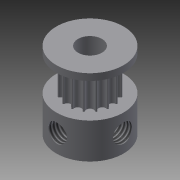
# Autodesk Inventor part: Pulley
Saved by Autodesk Inventor 2015 (Build 190159000, 159)
## iProperties
Created: 2017-01-19
Part Number: Pulley
Material: Generic
Document SubType Name: Modeling
Designer: Ernest
Density: 1 g/cm^3
Appearance: Default
Mass: 1.3342 g
Surface Area: 14.8455 cm^2
Volume: 1.3342 cm^3
Author: Ernest
Autodesk Inventor part; units mm, degrees
ref_plane "YZ Plane" through (0, 0, 0) normal (1, 0, 0) x (0, 1, 0)
ref_plane "XZ Plane" through (0, 0, 0) normal (0, 1, 0) x (-1, 0, 0)
ref_plane "XY Plane" through (0, 0, 0) normal (0, 0, 1) x (1, 0, 0)
sketch "Sketch1" plane through (0, 0, 0) normal (0, 0, 1) x (1, 0, 0)
  arc A0 (-0.7443, 4.7926) -> (-1.1464, 4.7126) centre (0, 0) ccw
  line L0 (0, 0) -> (0, 4.7) construction
  arc A1 (-0.7443, 4.7926) -> (0.7443, 4.7926) centre (0, 4.7) ccw
  arc A2 (-2.5216, 4.1429) -> (-1.1464, 4.7126) centre (-1.7986, 4.3422) ccw
  arc A3 (-3.9151, 2.8626) -> (-2.8626, 3.9151) centre (-3.3234, 3.3234) ccw
  arc A4 (-4.7126, 1.1464) -> (-4.1429, 2.5216) centre (-4.3422, 1.7986) ccw
  arc A5 (-4.7926, -0.7443) -> (-4.7926, 0.7443) centre (-4.7, 0) ccw
  arc A6 (-4.1429, -2.5216) -> (-4.7126, -1.1464) centre (-4.3422, -1.7986) ccw
  arc A7 (-2.8626, -3.9151) -> (-3.9151, -2.8626) centre (-3.3234, -3.3234) ccw
  arc A8 (-1.1464, -4.7126) -> (-2.5216, -4.1429) centre (-1.7986, -4.3422) ccw
  arc A9 (0.7443, -4.7926) -> (-0.7443, -4.7926) centre (0, -4.7) ccw
  arc A10 (2.5216, -4.1429) -> (1.1464, -4.7126) centre (1.7986, -4.3422) ccw
  arc A11 (3.9151, -2.8626) -> (2.8626, -3.9151) centre (3.3234, -3.3234) ccw
  arc A12 (4.7126, -1.1464) -> (4.1429, -2.5216) centre (4.3422, -1.7986) ccw
  arc A13 (4.7926, 0.7443) -> (4.7926, -0.7443) centre (4.7, 0) ccw
  arc A14 (4.1429, 2.5216) -> (4.7126, 1.1464) centre (4.3422, 1.7986) ccw
  arc A15 (2.8626, 3.9151) -> (3.9151, 2.8626) centre (3.3234, 3.3234) ccw
  arc A16 (1.1464, 4.7126) -> (2.5216, 4.1429) centre (1.7986, 4.3422) ccw
  arc A17 (1.1464, 4.7126) -> (0.7443, 4.7926) centre (0, 0) ccw
  arc A18 (2.8626, 3.9151) -> (2.5216, 4.1429) centre (0, 0) ccw
  arc A19 (4.1429, 2.5216) -> (3.9151, 2.8626) centre (0, 0) ccw
  arc A20 (4.7926, 0.7443) -> (4.7126, 1.1464) centre (0, 0) ccw
  arc A21 (4.7126, -1.1464) -> (4.7926, -0.7443) centre (0, 0) ccw
  arc A22 (3.9151, -2.8626) -> (4.1429, -2.5216) centre (0, 0) ccw
  arc A23 (2.5216, -4.1429) -> (2.8626, -3.9151) centre (0, 0) ccw
  arc A24 (0.7443, -4.7926) -> (1.1464, -4.7126) centre (0, 0) ccw
  arc A25 (0, -4.85) -> (0.7443, -4.7926) centre (0, 0) ccw
  arc A26 (-1.1464, -4.7126) -> (-0.7443, -4.7926) centre (0, 0) ccw
  arc A27 (-2.8626, -3.9151) -> (-2.5216, -4.1429) centre (0, 0) ccw
  arc A28 (-4.1429, -2.5216) -> (-3.9151, -2.8626) centre (0, 0) ccw
  arc A29 (-4.7926, -0.7443) -> (-4.7126, -1.1464) centre (0, 0) ccw
  arc A30 (-4.7126, 1.1464) -> (-4.7926, 0.7443) centre (0, 0) ccw
  arc A31 (-3.9151, 2.8626) -> (-4.1429, 2.5216) centre (0, 0) ccw
  arc A32 (-2.5216, 4.1429) -> (-2.8626, 3.9151) centre (0, 0) ccw
  dimension "d0" = 9.7
  dimension "d1" = 4.7
  dimension "d2" = 1.5
  dimension "d5" = 360
  constraints: 66 point on circle, 33 centre point, 2 coincident, 2 end point, 1 point on line, 1 vertical, 65 other
  measures "d0" diameter of A0
  measures "d1" distance of L0.start L0.end
  measures "d2" diameter of A1
extrude "Extrusion1" add sketch "Sketch1" along normal blind 7.15
fillet "Fillet1" radius 0.14 32 edges at (-0.7443, 4.7926, 3.575) (-1.1464, 4.7126, 3.575) (0.7443, 4.7926, 3.575) (1.1464, 4.7126, 3.575) (2.5216, 4.1429, 3.575) (2.8626, 3.9151, 3.575) (-2.5216, 4.1429, 3.575) (-2.8626, 3.9151, 3.575) (-3.9151, 2.8626, 3.575) (-4.1429, 2.5216, 3.575) (-4.7126, 1.1464, 3.575) (-4.7926, 0.7443, 3.575) (-4.7926, -0.7443, 3.575) (-4.7126, -1.1464, 3.575) (-4.1429, -2.5216, 3.575) (-3.9151, -2.8626, 3.575) (-2.8626, -3.9151, 3.575) (-2.5216, -4.1429, 3.575) (-0.7443, -4.7926, 3.575) (-1.1464, -4.7126, 3.575) (0.7443, -4.7926, 3.575) (1.1464, -4.7126, 3.575) (2.8626, -3.9151, 3.575) (2.5216, -4.1429, 3.575) (3.9151, -2.8626, 3.575) (4.1429, -2.5216, 3.575) (4.7126, -1.1464, 3.575) (4.7926, -0.7443, 3.575) (4.7126, 1.1464, 3.575) (4.7926, 0.7443, 3.575) (4.1429, 2.5216, 3.575) (3.9151, 2.8626, 3.575)
sketch "Sketch2" plane through (0, 0, 7.15) normal (0, 0, 1) x (1, 0, 0)
  circle A0 centre (0, 0) radius 2.5
  circle A1 centre (0, 0) radius 7
  dimension "d10" = 5
  dimension "d11" = 14
  constraints: 2 centre point, 2 coincident
  measures "d10" diameter of A0
  measures "d11" diameter of A1
extrude "Extrusion2" add sketch "Sketch2" along normal blind 1.4
extrude "Extrusion3" cut sketch "Sketch2" against normal blind 10 contours A0
sketch "Sketch3" plane through (0, 0, 0) normal (0, 0, -1) x (-1, 0, 0)
  circle A0 centre (0, 0) radius 7
  circle A1 centre (0, 0) radius 2.5
  dimension "d16" = 14
  constraints: 2 centre point, 2 coincident
  measures "d16" diameter of A0
extrude "Extrusion4" add sketch "Sketch3" along normal blind 7.4
sketch "Sketch4" plane through (0, 0, 0) normal (1, 0, 0) x (0, 1, 0)
  line L0 (-7, -7.4) -> (7, -7.4) projected
  line L1 (7, 0) -> (-7, 0) projected
  line L2 (7, 0) -> (-7, 0) projected
  line L3 (4.7501, 0) -> (4.5704, 0) projected
  line L4 (4.7632, 0) -> (4.7501, 0) projected
  line L5 (4.6374, 0) -> (4.7632, 0) projected
  line L6 (4.6374, 0) -> (4.6374, 0) projected
  line L7 (4.7632, 0) -> (4.6374, 0) projected
  line L8 (4.7501, 0) -> (4.7632, 0) projected
  line L9 (4.5704, 0) -> (4.7501, 0) projected
  line L10 (3.9984, 0) -> (4.5704, 0) projected
  line L11 (4.0512, 0) -> (3.9984, 0) projected
  line L12 (4.0139, 0) -> (4.0512, 0) projected
  line L13 (3.8076, 0) -> (4.0139, 0) projected
  line L14 (2.7507, 0) -> (3.8076, 0) projected
  line L15 (2.7223, 0) -> (2.7507, 0) projected
  line L16 (2.6666, 0) -> (2.7223, 0) projected
  line L17 (2.4652, 0) -> (2.6666, 0) projected
  line L18 (1.0842, 0) -> (2.4652, 0) projected
  line L19 (0.9791, 0) -> (1.0842, 0) projected
  line L20 (0.9133, 0) -> (0.9791, 0) projected
  line L21 (0.7474, 0) -> (0.9133, 0) projected
  line L22 (-0.7474, 0) -> (0.7474, 0) projected
  line L23 (-0.9133, 0) -> (-0.7474, 0) projected
  line L24 (-0.9791, 0) -> (-0.9133, 0) projected
  line L25 (-1.0842, 0) -> (-0.9791, 0) projected
  line L26 (-2.4652, 0) -> (-1.0842, 0) projected
  line L27 (-2.6666, 0) -> (-2.4652, 0) projected
  line L28 (-2.7223, 0) -> (-2.6666, 0) projected
  line L29 (-2.7507, 0) -> (-2.7223, 0) projected
  line L30 (-3.8076, 0) -> (-2.7507, 0) projected
  line L31 (-4.0139, 0) -> (-3.8076, 0) projected
  line L32 (-4.0512, 0) -> (-4.0139, 0) projected
  line L33 (-3.9984, 0) -> (-4.0512, 0) projected
  line L34 (-4.5704, 0) -> (-3.9984, 0) projected
  line L35 (-4.7501, 0) -> (-4.5704, 0) projected
  line L36 (-4.7632, 0) -> (-4.7501, 0) projected
  line L37 (-4.6374, 0) -> (-4.7632, 0) projected
  line L38 (-4.6374, 0) -> (-4.6374, 0) projected
  line L39 (-4.7632, 0) -> (-4.6374, 0) projected
  line L40 (-4.7501, 0) -> (-4.7632, 0) projected
  line L41 (-4.5704, 0) -> (-4.7501, 0) projected
  line L42 (-3.9984, 0) -> (-4.5704, 0) projected
  line L43 (-4.0512, 0) -> (-3.9984, 0) projected
  line L44 (-4.0139, 0) -> (-4.0512, 0) projected
  line L45 (-3.8076, 0) -> (-4.0139, 0) projected
  line L46 (-2.7507, 0) -> (-3.8076, 0) projected
  line L47 (-2.7223, 0) -> (-2.7507, 0) projected
  line L48 (-2.6666, 0) -> (-2.7223, 0) projected
  line L49 (-2.4652, 0) -> (-2.6666, 0) projected
  line L50 (-1.0842, 0) -> (-2.4652, 0) projected
  line L51 (-0.9791, 0) -> (-1.0842, 0) projected
  line L52 (-0.9133, 0) -> (-0.9791, 0) projected
  line L53 (-0.7474, 0) -> (-0.9133, 0) projected
  line L54 (0.7474, 0) -> (-0.7474, 0) projected
  line L55 (0.9133, 0) -> (0.7474, 0) projected
  line L56 (0.9791, 0) -> (0.9133, 0) projected
  line L57 (1.0842, 0) -> (0.9791, 0) projected
  line L58 (2.4652, 0) -> (1.0842, 0) projected
  line L59 (2.6666, 0) -> (2.4652, 0) projected
  line L60 (2.7223, 0) -> (2.6666, 0) projected
  line L61 (2.7507, 0) -> (2.7223, 0) projected
  line L62 (3.8076, 0) -> (2.7507, 0) projected
  line L63 (4.0139, 0) -> (3.8076, 0) projected
  line L64 (4.0512, 0) -> (4.0139, 0) projected
  line L65 (3.9984, 0) -> (4.0512, 0) projected
  line L66 (4.5704, 0) -> (3.9984, 0) projected
  circle A0 centre (0, -3.7) radius 1.95
  point P0 (0, 0)
  dimension "d19" = 7.4
  dimension "d20" = 3.7
  dimension "d21" = 3.9
  constraints: 1 centre point
  measures "d19" distance from line of L0 point (0, 0)
  measures "d20" distance from line of L0 A0.centre
  measures "d21" diameter of A0
extrude "Extrusion5" cut sketch "Sketch4" along normal blind 7.4
thread "Thread1" size "M4x0.7" class "6H" standard "ANSI Metric M Profile" full length
pattern_circular "Circular Pattern1" count 2 over 90 about axis through (0, 0, -10) along (0, 0, -1) of "Extrusion5"
equation "\"d20\" = 0.5 * d19"
body "Solid1"
